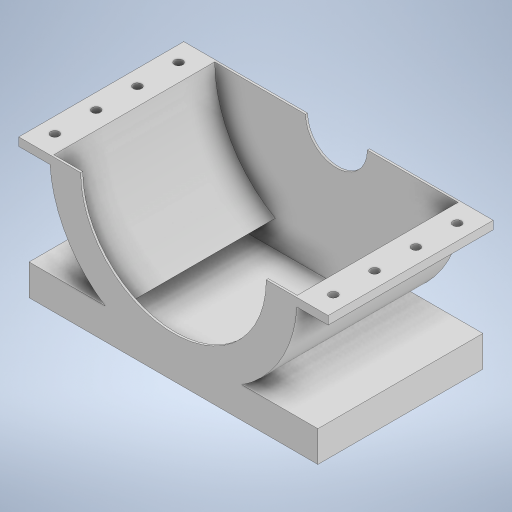
# Autodesk Inventor part: Carcaça Inferior do Motor Industiral
Saved by Autodesk Inventor 2023 (Build 270158030, 158C)
## iProperties
Created: 2022-07-19
Part Number: Carcaça Inferior do Motor Industiral
Material: Generic
Document SubType Name: Modeling
Designer: coqui
Density: 1 g/cm^3
Appearance: Default
Author: coqui
Autodesk Inventor part; units mm, degrees
ref_plane "YZ Plane" through (0, 0, 0) normal (1, 0, 0) x (0, 1, 0)
ref_plane "XZ Plane" through (0, 0, 0) normal (0, 1, 0) x (-1, 0, 0)
ref_plane "XY Plane" through (0, 0, 0) normal (0, 0, 1) x (1, 0, 0)
sketch "Sketch1" plane through (0, 0, 0) normal (0, 0, 1) x (1, 0, 0)
  line L0 (-60, 0) -> (60, 0)
  line L1 (70, -50) -> (70, -65)
  line L2 (70, -65) -> (-70, -65)
  line L3 (-70, -65) -> (-70, -50)
  line L4 (-70, -50) -> (70, -65) construction
  line L5 (-70, -50) -> (-33.1662, -50)
  line L6 (33.1662, -50) -> (70, -50)
  arc A0 (-60, 0) -> (-33.1662, -50) centre (0, 0) ccw
  arc A1 (33.1662, -50) -> (60, 0) centre (0, 0) ccw
  line L7 (70, -50) -> (24.1881, -54.9084) construction
  line L8 (0, -57.5) -> (-70, -65) construction
  dimension "d1" = 15
  dimension "d2" = 140
  dimension "d3" = 0
  dimension "d4" = 65
  constraints: 18 end point, 4 point on circle, 3 horizontal, 3 midpoint, 3 parallel, 2 centre point, 2 perpendicular, 1 coincident
  measures "d1" distance of L1.start L1.end
  measures "d2" distance of L3.end L1.start
  measures "d3" horizontal distance of point (0, 0) L8.start
  measures "d4" distance between parallel lines of L0 L2
extrude "Extrusion1" add sketch "Sketch1" along normal mid plane 80
shell "Shell1" thickness 1 removed faces 1 at (-20, 0, 13.3333)
sketch "Sketch2" plane through (0, 0, 40) normal (0, 0, 1) x (1, 0, 0)
  circle A0 centre (0, 0) radius 45
  dimension "d8" = 90
  constraints: 1 centre point, 1 coincident
  measures "d8" diameter of A0
extrude "Extrusion2" cut sketch "Sketch2" against normal blind 2
sketch "Sketch3" plane through (-69, -64, -39) normal (0, 0, 1) x (1, 0, 0)
  circle A0 centre (69, 64) radius 15
  dimension "d11" = 30
  constraints: 1 centre point, 1 coincident
  measures "d11" diameter of A0
extrude "Extrusion3" cut sketch "Sketch3" against normal blind 2
sketch "Sketch4" plane through (0, 0, 0) normal (0, 0, 1) x (1, 0, 0)
  line L0 (60, 0) -> (45, 0) projected
  line L1 (59.4, 0) -> (75, 0)
  line L2 (75, 0) -> (75, -4)
  line L3 (75, -4) -> (59.4, -4)
  line L4 (59.4, -4) -> (59.4, 0)
  line L5 (-70, -65) -> (70, -65) projected
  line L6 (0, 14.3485) -> (0, -121.7011) construction
  line L7 (-60, 0) -> (-45, 0)
  line L8 (-59.4, 0) -> (-75, 0)
  line L9 (-75, 0) -> (-75, -4)
  line L10 (-75, -4) -> (-59.4, -4)
  line L11 (-59.4, -4) -> (-59.4, 0)
  point P0 (0, 0)
  dimension "d14" = 65
  dimension "d15" = 4
  dimension "d16" = 15.6
  dimension "d17" = 75
  constraints: 20 end point, 6 symmetric about line, 2 parallel, 2 point on line, 1 horizontal, 1 perpendicular, 1 vertical
  measures "d14" distance between parallel lines of L5 L1
  measures "d15" distance of L1.end L2.end
  measures "d16" distance of L2.end L3.end
  measures "d17" distance from line of point (0, 0) L2
extrude "Extrusion4" add sketch "Sketch4" along normal mid plane 80
sketch "Sketch5" plane through (59.8665, -4, -40) normal (0, -1, 0) x (1, 0, 0)
  circle A0 centre (7.6335, 10) radius 2.05
  line L0 (15.1335, 0) -> (0, 0) projected
  line L1 (15.1335, 80) -> (15.1335, 0) projected
  circle A1 centre (7.6335, 30) radius 2.05
  circle A2 centre (7.6335, 50) radius 2.05
  circle A3 centre (7.6335, 70) radius 2.05
  circle A4 centre (-127.3665, 10) radius 2.05
  circle A5 centre (-127.3665, 30) radius 2.05
  circle A6 centre (-127.3665, 50) radius 2.05
  circle A7 centre (-127.3665, 70) radius 2.05
  point P0 (-59.8665, 40)
  point P1 (15.1335, 20)
  point P2 (15.1335, 40)
  point P3 (15.1335, 60)
  point P4 (-119.8665, 0)
  point P5 (-119.8665, 20)
  point P6 (-119.8665, 40)
  point P7 (-119.8665, 60)
  dimension "d20" = 4.1
  dimension "d21" = 10
  dimension "d22" = 7.5
  dimension "d25" = 20
  dimension "d28" = 135
  constraints: 8 centre point, 1 horizontal, 1 vertical, 21 other
  measures "d20" diameter of A0
  measures "d21" distance from line of L0 A0.centre
  measures "d22" distance from line of L1 A0.centre
  measures "d25" distance of A0.centre A1.centre
  measures "d28" distance of A0.centre A4.centre
extrude "Extrusion5" cut sketch "Sketch5" against normal blind 80
body "Solid1"
